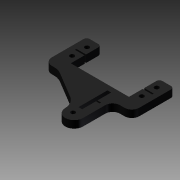
# Autodesk Inventor part: braket atas 2
Saved by Autodesk Inventor 2012 (Build 160160000, 160)
## iProperties
Created: 2011-10-02
Part Number: braket atas 2
Material: Default
Document SubType Name: Modeling
Designer: Yadi Irawan
Density: 1 g/cm^3
Author: Yadi Irawan
Autodesk Inventor part; units mm, degrees
ref_plane "YZ Plane" through (0, 0, 0) normal (1, 0, 0) x (0, 1, 0)
ref_plane "XZ Plane" through (0, 0, 0) normal (0, 1, 0) x (-1, 0, 0)
ref_plane "XY Plane" through (0, 0, 0) normal (0, 0, 1) x (1, 0, 0)
sketch "Sketch1" plane through (0, 0, 0) normal (0, 0, 1) x (1, 0, 0)
  line L0 (0, 0) -> (39.7, 0)
  circle A0 centre (43.66, 15) radius 1.5
  circle A1 centre (43.66, 4.8) radius 1.5
  circle A2 centre (-3.96, 15) radius 1.5
  circle A3 centre (-3.96, 4.8) radius 1.5
  line L1 (46.2, 9.9) -> (46.2, 10.4)
  line L2 (46.2, 10.4) -> (39.7, 10.4)
  line L3 (46.2, 9.9) -> (46.2, 9.4)
  line L4 (46.2, 9.4) -> (39.7, 9.4)
  line L5 (39.7, 0) -> (39.7, 9.4)
  line L6 (39.7, 10.4) -> (39.7, 18.8)
  line L7 (-6.5, 9.9) -> (-6.5, 10.4)
  line L8 (-6.5, 10.4) -> (0, 10.4)
  line L9 (-6.5, 9.4) -> (0, 9.4)
  line L10 (-6.5, 9.9) -> (-6.5, 9.4)
  line L11 (0, 9.4) -> (0, 0)
  line L12 (29.8, -3.5) -> (31.05, -3.5)
  line L13 (31.05, -23.3) -> (28.55, -23.3)
  line L14 (28.55, -23.3) -> (28.55, -3.5)
  line L15 (28.55, -3.5) -> (29.8, -3.5)
  line L16 (29.8, -23.3) -> (29.8, -28.3)
  circle A4 centre (29.8, -28.3) radius 1.5
  line L17 (31.05, -23.3) -> (31.05, -13.9)
  line L18 (31.05, -13.9) -> (33.55, -13.9)
  line L19 (33.55, -13.9) -> (33.55, -12.9)
  line L20 (33.55, -12.9) -> (31.05, -12.9)
  line L21 (31.05, -12.9) -> (31.05, -3.5)
  line L22 (36.55, -14.9) -> (36.55, -28.3)
  line L23 (-10, 0) -> (-10, -3)
  line L24 (36.55, -13) -> (36.55, -14.9)
  line L25 (41.55, -8) -> (44.7, -8)
  line L26 (49.7, -3) -> (49.7, 0)
  arc A5 (24.55, -28.3) -> (36.55, -28.3) centre (30.55, -28.3) ccw
  arc A6 (44.7, -8) -> (49.7, -3) centre (44.7, -3) ccw
  arc A7 (-10, -3) -> (-5, -8) centre (-5, -3) ccw
  arc A8 (41.55, -8) -> (36.55, -13) centre (41.55, -13) ccw
  line L27 (24.55, -28.6619) -> (24.55, -28.3)
  line L28 (-3.2198, -8) -> (-5, -8)
  line L29 (1.9251, -9.4251) -> (19.695, -20.087)
  arc A9 (1.9251, -9.4251) -> (-3.2198, -8) centre (-3.2198, -18) ccw
  arc A10 (24.55, -28.6619) -> (19.695, -20.087) centre (14.55, -28.6619) ccw
  line L30 (-2, 20.8) -> (-8, 20.8)
  line L31 (-10, 18.8) -> (-10, 0)
  line L32 (41.7, 20.8) -> (47.7, 20.8)
  line L33 (49.7, 18.8) -> (49.7, 0)
  arc A11 (0, 18.8) -> (-2, 20.8) centre (-2, 18.8) ccw
  arc A12 (-8, 20.8) -> (-10, 18.8) centre (-8, 18.8) ccw
  arc A13 (41.7, 20.8) -> (39.7, 18.8) centre (41.7, 18.8) ccw
  arc A14 (49.7, 18.8) -> (47.7, 20.8) centre (47.7, 18.8) ccw
  line L34 (0, 18.8) -> (0, 10.4)
  point P0 (0, 20.8)
  point P1 (-10, 20.8)
  dimension "d13" = 1.25
  dimension "d15" = 2.5
  dimension "d16" = 19.8
  dimension "d17" = 5
  dimension "d25" = 9.4
  dimension "d26" = 2.5
  dimension "d27" = 1
  dimension "d28" = 1
  dimension "d29" = 1
  dimension "d30" = 6.5
  dimension "d48" = 5
  dimension "d54" = 10
  dimension "d57" = 10
  dimension "d58" = 2
  constraints: 70 end point, 20 point on circle, 15 centre point, 15 tangent, 6 equal radius, 4 coincident, 4 point on line, 1 midpoint, 1 perpendicular
  measures "d13" distance of L12.start L12.end
  measures "d15" distance of L13.start L13.end
  measures "d16" distance of L13.end L14.end
  measures "d17" distance of L16.start L16.end
  measures "d25" distance of L13.start L17.end
  measures "d26" distance of L17.end L18.end
  measures "d27" distance of L18.end L19.end
  measures "d28" distance of L4.start L1.end
  measures "d29" distance between parallel lines of L9 L8
  measures "d30" distance of L4.start L4.end
  measures "d48" radius of A6
  measures "d54" radius of A9
  measures "d57" distance of point (0, 20.8) point (-10, 20.8)
  measures "d58" radius of A11
extrude "Extrusion1" add sketch "Sketch1" along normal blind 5
body "Solid1"
